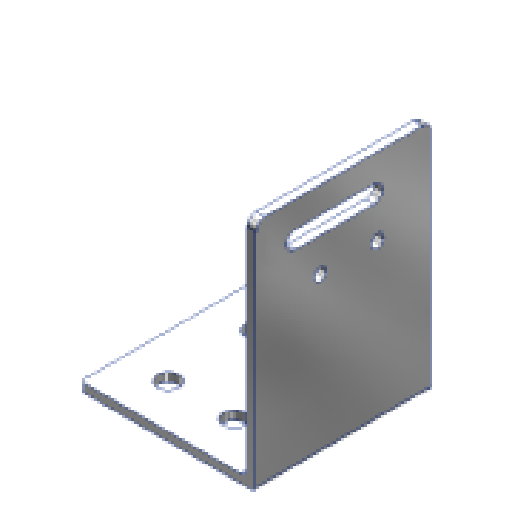
# Autodesk Inventor part: BRACKET_MOTOR
Saved by Autodesk Inventor 2025 (Build 290162000, 162)
## iProperties
Created: 2026-01-21
Part Number: BRACKET_MOTOR
Material: Aluminio 6061
Document SubType Name: Sheet Metal
Designer: HP
Density: 2.7 g/cm^3
Appearance: Aluminio - Plano
Sheet Metal Rule: Por defecto_mm
Author: HP
Autodesk Inventor part; units mm, degrees
ref_plane "YZ Plane" through (0, 0, 0) normal (1, 0, 0) x (0, 1, 0)
ref_plane "XZ Plane" through (0, 0, 0) normal (0, 1, 0) x (-1, 0, 0)
ref_plane "XY Plane" through (0, 0, 0) normal (0, 0, 1) x (1, 0, 0)
sketch "Boceto1" plane through (0, 0, 0) normal (1, 0, 0) x (0, 1, 0)
  line L0 (-6.321, 6.321) -> (6.321, 6.321) construction
  line L1 (6.321, 6.321) -> (6.321, -6.321) construction
  line L2 (6.321, -6.321) -> (-6.321, -6.321) construction
  line L3 (-6.321, -6.321) -> (-6.321, 6.321) construction
  line L4 (-6.321, 6.321) -> (6.321, -6.321) construction
  line L5 (6.321, 6.321) -> (-6.321, -6.321) construction
  circle A0 centre (6.321, -6.321) radius 0.875
  line L6 (0, 0) -> (7.9878, 0) construction
  circle A1 centre (6.321, 6.321) radius 0.875
  line L7 (0, 0) -> (0, -13.4562) construction
  circle A2 centre (-6.321, -6.321) radius 0.875
  circle A3 centre (-6.321, 6.321) radius 0.875
  circle A4 centre (0, 0) radius 5.5
  line L8 (10, 20) -> (-20, 20)
  line L9 (-20, 20) -> (-20, -20)
  line L10 (-20, -20) -> (10, -20)
  line L11 (10, -20) -> (10, 20)
  dimension "d0" = 12.642
  dimension "d1" = 12.642
  dimension "d2" = 1.75
  dimension "d3" = 11
  dimension "d4" = 30
  dimension "d6" = 20
  dimension "d7" = 10
  dimension "d26" = 20
  constraints: 24 end point, 5 centre point, 4 parallel, 3 coincident, 3 horizontal, 3 symmetric about line, 2 midpoint, 2 perpendicular, 1 vertical, 3 other
  measures "d0" distance of L1.end L2.end
  measures "d1" distance of L0.end L1.end
  measures "d2" diameter of A0
  measures "d3" diameter of A4
  measures "d4" distance of L10.end L9.end
  measures "d6" distance from line of L6.start L8
  measures "d7" distance from line of L6.start L11
  measures "d26" distance from line of L10 L6.start
extrude "Extrusión1" add sketch "Boceto1" along normal blind 2
sketch "Boceto2" plane through (0, -20, -20) normal (0, -1, 0) x (1, 0, 0)
  line L0 (2, 0) -> (2, 40) projected
  line L1 (2, 40) -> (-38, 40)
  line L2 (-38, 40) -> (-38, 0)
  line L3 (-38, 0) -> (2, 0)
  line L4 (2, 0) -> (2, 40)
  point P0 (0, 20)
  point P1 (2, 0)
  dimension "d10" = 40
  dimension "d11" = 40
  constraints: 8 end point, 2 parallel, 1 horizontal, 1 perpendicular
  measures "d10" distance of L3.end L2.end
  measures "d11" distance of L2.end L1.end
extrude "Extrusión2" add sketch "Boceto2" along normal blind 2
fillet "Empalme1" radius 1.5 1 edges at (0, -20, 0)
fillet "Empalme2" radius 1 5 edges at (1, 10, 20) (1, 10, -20) (-38, -21, 20) (-38, -21, -20) (2, -22, 0)
sketch "Boceto4" plane through (0, -20, -20) normal (0, 1, 0) x (1, 0, 0)
  circle A0 centre (-13, -10) radius 2.5
  circle A1 centre (-13, -30) radius 2.5
  circle A2 centre (-28, -10) radius 2.5
  circle A3 centre (-28, -30) radius 2.5
  line L0 (-1.5, -40) -> (-37, -40) projected
  line L1 (-38, -39) -> (-38, -1) projected
  point P0 (0, -20)
  dimension "d27" = 5
  dimension "d28" = 5
  dimension "d29" = 5
  dimension "d30" = 5
  dimension "d31" = 10
  dimension "d32" = 20
  dimension "d33" = 20
  dimension "d34" = 15
  dimension "d35" = 10
  constraints: 4 centre point, 2 vertical alignment, 1 horizontal alignment
  measures "d27" diameter of A0
  measures "d28" diameter of A1
  measures "d29" diameter of A2
  measures "d30" diameter of A3
  measures "d31" distance from line of A1.centre L0
  measures "d32" distance of A0.centre A1.centre
  measures "d33" distance of A2.centre A3.centre
  measures "d34" distance of A3.centre A1.centre
  measures "d35" distance from line of L1 A3.centre
extrude "Extrusión4" cut sketch "Boceto4" against normal through all
sketch "Boceto5" plane through (2, 0, 0) normal (1, 0, 0) x (0, 0, -1)
  line L0 (20, -21) -> (-20, -21) projected
  line L1 (20, 9) -> (20, -21) projected
  arc A0 (20, 9) -> (19, 10) centre (19, 9) ccw projected
  line L2 (19, 10) -> (-19, 10) projected
  arc A1 (-19, 10) -> (-20, 9) centre (-19, 9) ccw projected
  line L3 (-20, 9) -> (-20, -21) projected
  circle A2 centre (0, 0) radius 5.5 projected
  circle A3 centre (-6.321, -6.321) radius 0.875 projected
  circle A4 centre (6.321, -6.321) radius 0.875 projected
  circle A5 centre (-6.321, 6.321) radius 0.875 projected
  circle A6 centre (6.321, 6.321) radius 0.875 projected
extrude "Extrusión5" add sketch "Boceto5" against normal blind 2 contours A2 | A3 | A4 | A5 | A6
sketch "Boceto7" plane through (0, 0, 0) normal (-1, 0, 0) x (0, 0, 1)
  arc A0 (-19, 10) -> (-20, 9) centre (-19, 9) ccw projected
  line L0 (-20, -18.5) -> (-20, 9) projected
  line L1 (20, -18.5) -> (-20, -18.5) projected
  line L2 (20, 9) -> (20, -18.5) projected
  arc A1 (20, 9) -> (19, 10) centre (19, 9) ccw projected
  line L3 (-19, 10) -> (19, 10) projected
  line L4 (-20, -18.5) -> (20, -18.5)
  line L5 (20, -18.5) -> (20, 31.5)
  line L6 (20, 31.5) -> (-20, 31.5)
  line L7 (-20, 31.5) -> (-20, -18.5)
  point P0 (0, 0)
  dimension "d42" = 40
  dimension "d43" = 50
  constraints: 8 end point, 2 parallel, 1 horizontal, 1 perpendicular
  measures "d42" distance of L6.end L5.end
  measures "d43" distance of L5.end L4.end
extrude "Extrusión7" add sketch "Boceto7" against normal blind 2 contours A0 L7 L6 L5 A1 L3
fillet "Empalme3" radius 2 2 edges at (1, 31.5, -20) (1, 31.5, 20)
sketch "Boceto8" plane through (0, 0, 0) normal (-1, 0, 0) x (0, 0, 1)
  line L0 (-18, 31.5) -> (18, 31.5) construction
  line L1 (0, 31.5) -> (0, 13.8) construction
  line L2 (-20, -18.5) -> (-20, 29.5) construction
  line L3 (-20, 13.8) -> (19.9852, 13.8) construction
  line L4 (-20, 13.8) -> (-7.75, 13.8) construction
  circle A0 centre (-7.75, 13.8) radius 1.5
  circle A1 centre (5.25, 13.8) radius 1.5
  point P0 (0, 0)
  dimension "d47" = 17.7
  dimension "d48" = 12.25
  dimension "d49" = 3
  dimension "d50" = 3
  dimension "d51" = 13
  constraints: 6 end point, 3 point on line, 2 centre point, 1 coincident, 1 midpoint, 1 perpendicular, 1 vertical
  measures "d47" distance of L1.start L1.end
  measures "d48" distance of L3.start L4.end
  measures "d49" diameter of A0
  measures "d50" diameter of A1
  measures "d51" distance of L4.end A1.centre
extrude "Extrusión8" cut sketch "Boceto8" against normal blind 2
sketch "Boceto9" plane through (0, 0, 0) normal (-1, 0, 0) x (0, 0, 1)
  line L0 (-10, 23.5) -> (9, 23.5)
  line L1 (18, 31.5) -> (-18, 31.5) projected
  line L2 (9, 23.5) -> (-10, 23.5) construction
  line L3 (9, 25.5) -> (-10, 25.5)
  line L4 (-10, 21.5) -> (9, 21.5)
  arc A0 (9, 21.5) -> (9, 25.5) centre (9, 23.5) ccw
  arc A1 (-10, 25.5) -> (-10, 21.5) centre (-10, 23.5) ccw
  line L5 (-20, -18.5) -> (-20, 29.5) projected
  point P0 (0, 0)
  point P1 (0, 31.5)
  point P2 (0, 31.5)
  point P3 (-0.5, 23.5)
  dimension "d56" = 8
  dimension "d57" = 9
  dimension "d58" = 10
  dimension "d59" = 4
  constraints: 10 end point, 4 point on circle, 4 tangent, 3 midpoint, 2 centre point, 2 equal length, 1 horizontal
  measures "d56" distance between parallel lines of L0 L1
  measures "d57" horizontal distance of point (0, 31.5) L0.end
  measures "d58" horizontal distance of L0.start point (0, 31.5)
  measures "d59" diameter of A1
extrude "Extrusión9" cut sketch "Boceto9" against normal blind 2
sketch "Boceto11" plane through (0, 0, 0) normal (-1, 0, 0) x (0, 0, 1)
  circle A0 centre (0, 0) radius 5.5 projected
  circle A1 centre (5.25, 13.8) radius 1.5 projected
  dimension "d64" = 13.8
  measures "d64" vertical distance of A0.centre A1.centre
sketch "Boceto3" plane through (0, -20, -20) normal (0, 1, 0) x (1, 0, 0)
  line L0 (0, -40) -> (0, 0) projected
  line L1 (-28, 0) -> (0, 0) projected
  line L2 (-28, -40) -> (-28, 0) projected
  line L3 (0, -40) -> (-28, -40) projected
  line L4 (-6.125, -3.125) -> (-6.125, -36.875) construction
  line L5 (-7.25, -3.125) -> (-7.25, -36.875)
  line L6 (-5, -36.875) -> (-5, -3.125)
  arc A0 (-5, -3.125) -> (-7.25, -3.125) centre (-6.125, -3.125) ccw
  arc A1 (-7.25, -36.875) -> (-5, -36.875) centre (-6.125, -36.875) ccw
  line L7 (-21.875, -3.125) -> (-21.875, -36.875) construction
  line L8 (-23, -3.125) -> (-23, -36.875)
  line L9 (-20.75, -36.875) -> (-20.75, -3.125)
  arc A2 (-20.75, -3.125) -> (-23, -3.125) centre (-21.875, -3.125) ccw
  arc A3 (-23, -36.875) -> (-20.75, -36.875) centre (-21.875, -36.875) ccw
  point P0 (0, -20)
  point P1 (-6.125, -20)
  point P2 (-21.875, -20)
  point P3 (-21.875, -38)
  point P4 (-21.875, -2)
  point P5 (-6.125, -38)
  point P6 (-6.125, -2)
  dimension "d14" = 2.25
  dimension "d15" = 2.25
  dimension "d16" = 5
  dimension "d17" = 2
  dimension "d18" = 2
  dimension "d19" = 2
  dimension "d20" = 2
  dimension "d21" = 5
  constraints: 16 end point, 12 point on circle, 8 tangent, 4 centre point, 3 parallel, 2 midpoint, 1 vertical
  measures "d14" diameter of A1
  measures "d15" diameter of A3
  measures "d16" distance between parallel lines of L8 L2
  measures "d17" distance from line of L3 point (-21.875, -38)
  measures "d18" distance from line of L1 point (-21.875, -2)
  measures "d19" distance from line of L3 point (-6.125, -38)
  measures "d20" distance from line of L1 point (-6.125, -2)
  measures "d21" distance between parallel lines of L6 L0
equation "\"Radio_pliegue\" = Grosor"
equation "\"Anchura_desahogo_plegado\" = Grosor"
equation "\"Profundidad_desahogo_plegado\" = 0.5 * Grosor"
equation "\"Tamaño_destalonado\" = 4 * Grosor"
equation "\"Remanente_mínimo\" = 2 * Grosor"
equation "\"Radiodetransición\" = Radio_pliegue"
equation "\"Tamaño_de_radio_de_Jacobi\" = Radio_pliegue"
equation "\"TamañoSeparación\" = Grosor"
equation "\"Grosor\" = 2"
